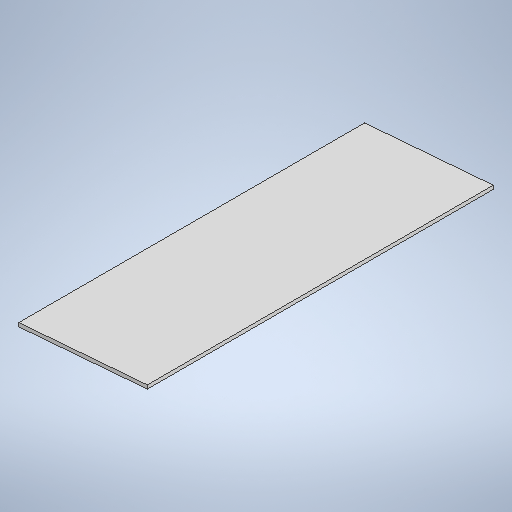
# Autodesk Inventor part: a
Saved by Autodesk Inventor 2025.2 (Build 292293000, 293)
## iProperties
Created: 2026-02-05
Part Number: a
Material: Generic
Document SubType Name: Modeling
Designer: Joefi
Density: 1 g/cm^3
Appearance: Default
Author: Joefi
Autodesk Inventor part; units mm, degrees
ref_plane "YZ Plane" through (0, 0, 0) normal (1, 0, 0) x (0, 1, 0)
ref_plane "XZ Plane" through (0, 0, 0) normal (0, 1, 0) x (-1, 0, 0)
ref_plane "XY Plane" through (0, 0, 0) normal (0, 0, 1) x (1, 0, 0)
sketch "Sketch1" plane through (0, 0, 0) normal (0, 1, 0) x (-1, 0, 0)
  line L0 (12.0423, -36.5791) -> (12.0423, 39.2223)
  line L1 (12.0423, 39.2223) -> (-13.874, 36.9549)
  line L2 (-13.874, 36.9549) -> (-13.874, -38.8464)
  line L3 (-13.874, -38.8464) -> (12.0423, -36.5791)
  line L4 (10.0423, 31.5831) -> (10.0423, -30.1647)
  arc A0 (5.4781, -35.1457) -> (10.0423, -30.1647) centre (5.0423, -30.1647) ccw
  line L5 (5.4781, -35.1457) -> (-6.4382, -36.1883)
  arc A1 (-11.874, -31.2073) -> (-6.4382, -36.1883) centre (-6.874, -31.2073) ccw
  line L6 (-11.874, -31.2073) -> (-11.874, 30.5406)
  arc A2 (-7.3097, 35.5216) -> (-11.874, 30.5406) centre (-6.874, 30.5406) ccw
  line L7 (-7.3097, 35.5216) -> (4.6065, 36.5641)
  arc A3 (10.0423, 31.5831) -> (4.6065, 36.5641) centre (5.0423, 31.5831) ccw
  line L8 (11.8423, -36.3958) -> (-13.674, -38.6282)
  line L9 (-13.674, -38.6282) -> (-13.674, 36.7717)
  line L10 (-13.674, 36.7717) -> (11.8423, 39.004)
  point P0 (0, 0)
  constraints: 22 end point, 8 point on circle, 4 centre point, 2 other
extrude "Extrusion1" add sketch "Sketch1" along normal blind 0.8 contours L3 L2 L1 L0 | L4 A0 L5 A1 L6 A2 L7 A3
body "Solid1"
